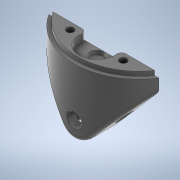
# Autodesk Inventor part: SplitBracketNut
Saved by Autodesk Inventor 2020 (Build 240168000, 168)
## iProperties
Created: 2019-05-28
Part Number: SplitBracketNut
Material: ABS Plastic
Document SubType Name: Modeling
Designer: Connor
Density: 1.06 g/cm^3
Appearance: Smooth - Black
Author: Connor
Autodesk Inventor part; units mm, degrees
ref_plane "YZ Plane" through (0, 0, 0) normal (1, 0, 0) x (0, 1, 0)
sketch "Sketch1" plane through (0, 0, 0) normal (0, 0, 1) x (1, 0, 0)
  line L0 (0, 0) -> (46.99, 0)
  line L1 (46.99, 0) -> (46.99, 47.625)
  line L2 (46.99, 47.625) -> (0, 47.625)
  line L3 (0, 47.625) -> (0, 0)
  line L4 (0, 47.625) -> (44.45, 47.625)
  line L5 (44.45, 47.625) -> (44.45, 50.8)
  line L6 (44.45, 50.8) -> (0, 50.8)
  line L7 (0, 50.8) -> (0, 47.625)
  circle A0 centre (0, 12.7) radius 12.7
  circle A1 centre (0, 12.7) radius 6.35
  line L8 (46.99, 47.625) -> (9.6065, 4.3931)
  line L9 (0, 0) -> (-46.99, 0)
  line L10 (-46.99, 0) -> (-46.99, 47.625)
  line L11 (-46.99, 47.625) -> (0, 47.625)
  line L12 (0, 47.625) -> (0, 0)
  line L13 (-46.99, 47.625) -> (-9.6065, 4.3931)
  dimension "d2" = 44.45
  dimension "d3" = 3.175
  dimension "d4" = 2.54
  dimension "d5" = 12.7
  dimension "d7" = 6.35
  dimension "d38" = 38.1
  constraints: 28 end point, 6 parallel, 3 horizontal, 3 perpendicular, 3 point on circle, 2 centre point, 2 equal length, 2 tangent, 1 coincident, 1 point on line
  measures "d2" distance of L6.end L5.end
  measures "d3" distance of L5.end L4.end
  measures "d4" distance between parallel lines of L5 L1
  measures "d5" diameter of A1
  measures "d7" radial gap between concentric circles of A1 A0
  measures "d38" distance from line of L6 A0.centre
revolve "Revolution1" add sketch "Sketch1" angle 180 about axis through (0, 47.625, 0) along (0, -1, 0) picked at (10.4113, 11.2324) picked at (2.0636, 13.171) contours A0 L8 L1 L0 | L3 A1 A0 | L3 A1 | A0 L3 L2 L8 | L2 L7 L6 L5
sketch "Sketch2" plane through (0, 0, 0) normal (1, 0, 0) x (0, 1, 0)
  line L0 (0, 0) -> (47.625, 0) projected
  line L1 (50.8, 44.45) -> (50.8, 0) projected
  line L2 (0, 0) -> (50.8, 0)
  line L3 (50.8, 0) -> (50.8, 25.4)
  line L4 (50.8, 25.4) -> (0, 25.4)
  line L5 (0, 25.4) -> (0, 0)
  dimension "d10" = 25.4
  constraints: 8 end point, 2 parallel, 1 horizontal, 1 perpendicular, 1 point on line
  measures "d10" distance between parallel lines of L0 L4
extrude "Extrusion1" cut sketch "Sketch2" along normal through all both and the other way through all
extrude "Extrusion3" cut sketch "Sketch1" along normal through all contours A0 L8 L1 L0 | L9 L10 L13 A0
sketch "Sketch8" plane through (0, 50.8, 0) normal (0, 1, 0) x (1, 0, 0)
  circle A0 centre (0, -30.48) radius 12.7
  point P0 (0, 0)
  dimension "d42" = 25.4
  dimension "d43" = 30.48
  constraints: 1 centre point, 1 vertical alignment
  measures "d42" diameter of A0
  measures "d43" distance of point (0, 0) A0.centre
extrude "Extrusion6" cut sketch "Sketch8" against normal blind 6.35
ref_plane "Work Plane3" through (0, 0, 0) normal (0, 1, 0) x (-1, 0, 0)
sketch "Sketch9" plane through (0, 0, 0) normal (0, 1, 0) x (-1, 0, 0)
  line L0 (-19.05, 30.48) -> (0, 0) construction
  line L1 (0, 0) -> (19.05, 30.48) construction
  dimension "d46" = 30.48
  dimension "d47" = 38.1
  constraints: 4 end point, 1 equal length, 1 horizontal alignment
  measures "d46" vertical distance of L0.end L0.start
  measures "d47" distance of L1.end L0.start
hole "Hole3" at (19.05, 0, 30.48) at (-19.05, 0, 30.48) direction (0, 1, 0) diameter 5.1594 end through all counterbore diameter 7.9375 counterbore depth 25.4
sketch "Sketch10" plane through (39.5335, 47.625, 25.4) normal (0, 0, -1) x (-1, 0, 0)
  arc A0 (29.927, -43.2319) -> (49.14, -43.2319) centre (39.5335, -34.925) ccw projected
  point P0 (39.5335, -47.625)
  constraints: 1 coincident
hole "Hole4" at (0, 12.7, 25.4) direction (0, 0, 1) diameter 9.525 end through all counterbore diameter 12.7 counterbore depth 6.35
ref_plane "Work Plane4" through (0, 12.7, 34.925) normal (0, 0, -1) x (-1, 0, 0)
sketch "Sketch14" plane through (0, 12.7, 34.925) normal (0, 0, -1) x (-1, 0, 0)
  circle A0 centre (0, 0) radius 4.7625 projected
  line L0 (0, 8.2489) -> (7.1437, 4.1244)
  line L1 (7.1437, 4.1244) -> (7.1437, -4.1244)
  line L2 (7.1437, -4.1244) -> (0, -8.2489)
  line L3 (0, -8.2489) -> (-7.1437, -4.1244)
  line L4 (-7.1437, -4.1244) -> (-7.1438, 4.1244)
  line L5 (-7.1438, 4.1244) -> (0, 8.2489)
  point P0 (0, -12.7)
  dimension "d68" = 14.2875
  constraints: 12 end point, 1 coincident, 1 vertical alignment, 13 other
  measures "d68" distance between parallel lines of L3 L0
extrude "Extrusion9" cut sketch "Sketch14" against normal blind 6.35
sketch "Sketch15" plane through (0, 0, 0) normal (0, 1, 0) x (-1, 0, 0)
  line L0 (7.1438, 34.925) -> (7.1438, 41.275) projected
  line L1 (0, 34.925) -> (7.1438, 34.925) projected
  line L2 (-7.1437, 34.925) -> (0, 34.925) projected
  line L3 (0, 41.275) -> (-7.1437, 41.275) projected
  line L4 (7.1438, 41.275) -> (0, 41.275) projected
  line L5 (-7.1437, 34.925) -> (-7.1437, 41.275) projected
  point P0 (0, 0)
extrude "Extrusion10" cut sketch "Sketch15" along normal up to surface (8.5756 mm away)
sketch "Sketch16" plane through (0, 44.45, 0) normal (0, 1, 0) x (1, 0, 0)
  arc A0 (-11.6397, -25.4) -> (11.6397, -25.4) centre (0, -30.48) ccw projected
  circle A1 centre (0, -30.48) radius 4.7625
  point P0 (0, 0)
  dimension "d73" = 9.525
  constraints: 1 centre point, 1 coincident
  measures "d73" diameter of A1
extrude "Extrusion11" cut sketch "Sketch16" against normal blind 3.175
fillet "Fillet1" radius 0.7937 7 edges at (19.05, 15.3139, 34.4488) (0, 0, 34.925) (7.1437, 2.1997, 38.1) (0, 0, 41.275) (-7.1438, 2.1997, 38.1) (-19.05, 15.3139, 34.4488) (-0.0367, 7.9376, 46.99)
fillet "Fillet2" radius 3.175 8 edges at (8.4739, 3.2404, 46.2196) (3.888, 0.6098, 46.8289) (-3.8823, 0.608, 46.8293) (-8.4809, 3.2467, 46.2183) (-26.6411, 24.0927, 38.708) (26.6411, 24.0927, 38.708) (-11.6397, 47.625, 25.4) (11.6397, 47.625, 25.4)
body "Solid1"
